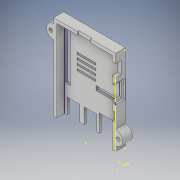
# Autodesk Inventor part: Oberteil_fertig2
Saved by Autodesk Inventor 2017 (Build 210142000, 142)
## iProperties
Part Number: Oberteil_fertig2
Material: Generisch
Document SubType Name: Modeling
Designer: Fynn
Density: 1 g/cm^3
Appearance: Vorgabe
Author: Fynn
Autodesk Inventor part; units mm, degrees
ref_plane "YZ Plane" through (0, 0, 0) normal (1, 0, 0) x (0, 1, 0)
ref_plane "XZ Plane" through (0, 0, 0) normal (0, 1, 0) x (-1, 0, 0)
ref_plane "XY Plane" through (0, 0, 0) normal (0, 0, 1) x (1, 0, 0)
sketch "Skizze1" plane through (0, 0, 0) normal (0, 1, 0) x (-1, 0, 0)
  line L0 (64.3291, 15.6705) -> (64.3291, 102.6705)
  line L1 (64.3291, 102.6705) -> (5.4791, 102.6705)
  line L2 (61.5291, 32.1705) -> (48.0291, 32.1705)
  line L3 (48.0291, 32.1705) -> (48.0291, 15.6705)
  line L4 (61.5291, 15.6705) -> (61.5291, 32.1705)
  line L5 (43.5291, 32.1705) -> (30.0291, 32.1705)
  line L6 (30.0291, 32.1705) -> (30.0291, 15.6705)
  line L7 (30.0291, 15.6705) -> (30.7791, 15.6705)
  line L8 (43.5291, 15.6705) -> (43.5291, 32.1705)
  line L9 (27.5291, 34.6705) -> (9.9291, 34.6705)
  line L10 (9.9291, 34.6705) -> (9.9291, 15.6705)
  line L11 (27.5291, 15.6705) -> (27.5291, 34.6705)
  line L12 (30.7791, 58.1705) -> (5.4791, 58.1705)
  line L13 (5.4791, 53.6705) -> (30.7791, 53.6705)
  line L14 (30.7791, 53.6705) -> (30.7791, 58.1705)
  line L15 (5.4791, 102.6705) -> (5.4791, 58.1705)
  line L16 (5.4791, 53.6705) -> (5.4791, 15.6705)
  line L17 (43.5291, 15.6705) -> (48.0291, 15.6705)
  line L18 (61.5291, 15.6705) -> (64.3291, 15.6705)
  line L19 (50.9791, 78.7705) -> (30.9791, 78.7705)
  line L20 (30.9791, 78.7705) -> (30.9791, 76.7705)
  line L21 (30.9791, 76.7705) -> (50.9791, 76.7705)
  line L22 (50.9791, 76.7705) -> (50.9791, 78.7705)
  line L23 (50.9791, 73.7705) -> (30.9791, 73.7705)
  line L24 (30.9791, 73.7705) -> (30.9791, 71.7705)
  line L25 (30.9791, 71.7705) -> (50.9791, 71.7705)
  line L26 (50.9791, 71.7705) -> (50.9791, 73.7705)
  line L27 (50.9791, 68.7705) -> (30.9791, 68.7705)
  line L28 (30.9791, 68.7705) -> (30.9791, 66.7705)
  line L29 (30.9791, 66.7705) -> (50.9791, 66.7705)
  line L30 (50.9791, 66.7705) -> (50.9791, 68.7705)
  line L31 (50.9791, 63.7705) -> (30.9791, 63.7705)
  line L32 (30.9791, 63.7705) -> (30.9791, 61.7705)
  line L33 (30.9791, 61.7705) -> (50.9791, 61.7705)
  line L34 (50.9791, 61.7705) -> (50.9791, 63.7705)
  line L35 (5.4791, 15.6705) -> (9.9291, 15.6705)
  line L36 (27.5291, 15.6705) -> (30.0291, 15.6705)
  line L37 (5.4791, 58.1705) -> (5.4791, 63.7705)
  line L38 (62.9791, 94.6705) -> (57.4791, 94.6705)
  line L39 (57.4791, 94.6705) -> (57.4791, 41.6705)
  line L40 (57.4791, 41.6705) -> (62.9791, 41.6705)
  line L41 (62.9791, 41.6705) -> (62.9791, 94.6705)
  dimension "d2" = 13.5
  dimension "d3" = 13.5
  dimension "d45" = 2.8
  dimension "d46" = 4.5
  dimension "d47" = 2.5
  dimension "d49" = 42.5
  dimension "d51" = 49
  dimension "d60" = 53
  dimension "d61" = 8
  dimension "d62" = 5.5
  dimension "d63" = 1.35
  dimension "d70" = 87
  dimension "d71" = 87
  dimension "d107" = 4.45
  dimension "d108" = 38
  dimension "d110" = 17.6
  dimension "d141" = 25.3
  dimension "d142" = 19
  constraints: 84 end point, 22 parallel, 13 horizontal, 13 perpendicular, 4 point on line
  measures "d2" distance of L2.start L2.end
  measures "d3" distance of L5.start L5.end
  measures "d45" distance of L4.start L0.start
  measures "d46" distance of L8.start L3.end
  measures "d47" distance of L11.start L6.end
  measures "d49" distance between parallel lines of L35 L12
  measures "d51" distance between parallel lines of L1 L13
  measures "d60" distance of L40.end L38.start
  measures "d61" distance between parallel lines of L1 L38
  measures "d62" distance of L38.start L38.end
  measures "d63" distance between parallel lines of L0 L41
  measures "d70" distance of L0.start L0.end
  measures "d71" distance of L16.end L1.end
  measures "d107" distance of L16.end L10.end
  measures "d108" distance of L13.start L16.end
  measures "d110" distance of L9.start L9.end
  measures "d141" distance between parallel lines of L14 L15
  measures "d142" distance between parallel lines of L13 L9
sketch "Skizze2" plane through (0, 0, 0) normal (0, 1, 0) x (-1, 0, 0)
  point P0 (0, 0)
extrude "Extrusion1" add sketch "Skizze1" along normal blind 3.5 contours L18 L4 L2 L3 L17 L8 L5 L6 L36 L11 L9 L10 L35 L16 L13 L14 L12 L15 L1 L0 | L41 L40 L39 L38
sketch "Skizze3" plane through (0, 0, 0) normal (0, -1, 0) x (1, 0, 0)
  line L0 (-9.9291, 15.6705) -> (-5.4791, 15.6705) projected
  line L1 (-64.3291, 102.6705) -> (-5.4791, 102.6705) projected
  line L2 (-5.4791, 15.6705) -> (-5.4791, 102.6705)
  line L3 (-5.4791, 102.6705) -> (-64.3291, 102.6705)
  line L4 (-64.3291, 102.6705) -> (-64.3291, 15.6705)
  point P0 (0, 0)
  constraints: 6 end point, 1 collinear, 1 perpendicular
sketch "Skizze4" plane through (0, 0, 0) normal (0, -1, 0) x (1, 0, 0)
  line L0 (-30.7791, 53.6705) -> (-5.4791, 53.6705) projected
  line L1 (-5.4791, 53.6705) -> (-5.4791, 15.6705) projected
  line L2 (-5.4791, 15.6705) -> (-5.4791, 102.6705)
  line L3 (-64.3291, 102.6705) -> (-5.4791, 102.6705) projected
  line L4 (-5.4791, 102.6705) -> (-64.3291, 102.6705)
  line L5 (-61.5291, 15.6705) -> (-64.3291, 15.6705) projected
  line L6 (-64.3291, 102.6705) -> (-64.3291, 15.6705)
  point P0 (0, 0)
  point P1 (-5.4791, 68.3705)
  point P2 (-5.4791, 63.3705)
  constraints: 6 end point, 2 perpendicular, 1 vertical, 1 other
sketch "Skizze5" plane through (0, 3.5, 0) normal (0, 1, 0) x (1, 0, 0)
  point P0 (0, 0)
sketch "Skizze6" plane through (0, 3.5, 0) normal (0, 1, 0) x (1, 0, 0)
  point P0 (0, 0)
sketch "Skizze7" plane through (0, 3.5, 0) normal (0, 1, 0) x (1, 0, 0)
  point P0 (0, 0)
sketch "Skizze8" plane through (0, 3.5, 0) normal (0, 1, 0) x (1, 0, 0)
  point P0 (0, 0)
sketch "Skizze9" plane through (0, 3.5, 0) normal (0, 1, 0) x (1, 0, 0)
  point P0 (0, 0)
sketch "Skizze10" plane through (0, 3.5, 0) normal (0, 1, 0) x (1, 0, 0)
  line L0 (-57.8291, -44.6705) -> (-63.3291, -44.6705)
  line L1 (-63.3291, -44.6705) -> (-63.3291, -95.6705)
  line L2 (-63.3291, -95.6705) -> (-57.8291, -95.6705)
  line L3 (-57.8291, -95.6705) -> (-57.8291, -44.6705)
  line L4 (-64.3291, -102.6705) -> (-5.4791, -102.6705) projected
  line L5 (-64.3291, -15.6705) -> (-64.3291, -102.6705) projected
  point P0 (0, 0)
  dimension "d64" = 51
  dimension "d65" = 5.5
  dimension "d66" = 7
  dimension "d67" = 1
  constraints: 8 end point, 2 parallel, 1 horizontal, 1 perpendicular
  measures "d64" distance of L2.end L0.start
  measures "d65" distance of L0.start L0.end
  measures "d66" distance between parallel lines of L4 L2
  measures "d67" distance between parallel lines of L5 L1
extrude "Extrusion2" cut sketch "Skizze10" against normal through all
sketch "Skizze11" plane through (0, 3.5, 0) normal (0, 1, 0) x (1, 0, 0)
  line L0 (-64.3291, -102.6705) -> (-64.3291, -15.6705) projected
  line L1 (-64.3291, -15.6705) -> (-64.3291, -102.6705) projected
  line L2 (-64.3291, -15.6705) -> (-67.8291, -15.6705)
  line L3 (-67.8291, -15.6705) -> (-67.8291, -106.1705)
  line L4 (-67.8291, -106.1705) -> (-1.9791, -106.1705)
  line L5 (-1.9791, -106.1705) -> (-1.9791, -15.6705)
  line L6 (-1.9791, -15.6705) -> (-5.4791, -15.6705)
  line L7 (-64.3291, -102.6705) -> (-5.4791, -102.6705) projected
  line L8 (-5.4791, -102.6705) -> (-64.3291, -102.6705)
  line L9 (-64.3291, -102.6705) -> (-64.3291, -15.6705)
  line L10 (-64.3291, -15.6705) -> (-64.3291, -102.6705)
  line L11 (-5.4791, -53.6705) -> (-5.4791, -15.6705) projected
  line L12 (-5.4791, -102.6705) -> (-5.4791, -15.6705)
  line L13 (-5.4791, -15.6705) -> (-1.9791, -15.6705)
  point P0 (0, 0)
  dimension "d77" = 3.5
  dimension "d78" = 3.5
  dimension "d79" = 3.5
  constraints: 20 end point, 6 perpendicular, 2 horizontal, 1 point on line, 1 vertical
  measures "d77" distance of L0.end L2.end
  measures "d78" distance of L5.end L6.end
  measures "d79" distance between parallel lines of L7 L4
sketch "Skizze12" plane through (0, 0, 0) normal (0, -1, 0) x (1, 0, 0)
  line L0 (-5.4791, 15.6705) -> (-9.9291, 15.6705) projected
  line L1 (-5.4791, 102.6705) -> (-5.4791, 58.1705) projected
  line L2 (-5.4791, 15.6705) -> (-5.4791, 102.6705)
  line L3 (-5.4791, 102.6705) -> (-64.3291, 102.6705)
  line L4 (-64.3291, 102.6705) -> (-64.3291, 15.6705)
  point P0 (0, 0)
  constraints: 6 end point, 2 perpendicular, 1 vertical
extrude "Extrusion3" add sketch "Skizze11" against normal blind 11.6
sketch "Skizze13" plane through (0, 3.5, 0) normal (0, 1, 0) x (1, 0, 0)
  line L0 (-67.8291, -15.6705) -> (-67.8291, -106.1705) projected
  arc A0 (-67.8291, -85.6705) -> (-67.8291, -100.6705) centre (-67.8291, -93.1705) ccw
  arc A1 (-67.8291, -21.1705) -> (-67.8291, -36.1705) centre (-67.8291, -28.6705) ccw
  arc A2 (-1.9791, -36.1705) -> (-1.9791, -21.1705) centre (-1.9791, -28.6705) ccw
  arc A3 (-1.9791, -100.6705) -> (-1.9791, -85.6705) centre (-1.9791, -93.1705) ccw
  line L1 (-67.8291, -106.1705) -> (-1.9791, -106.1705) projected
  line L2 (-1.9791, -15.6705) -> (-9.9291, -15.6705) projected
  line L3 (-1.9791, -106.1705) -> (-1.9791, -15.6705) projected
  point P0 (0, 0)
  dimension "d82" = 15
  dimension "d83" = 15
  dimension "d84" = 15
  dimension "d85" = 15
  dimension "d86" = 13
  dimension "d87" = 13
  dimension "d88" = 13
  dimension "d89" = 13
  constraints: 10 point on line, 8 point on circle, 4 centre point
  measures "d82" diameter of A0
  measures "d83" diameter of A1
  measures "d84" diameter of A2
  measures "d85" diameter of A3
  measures "d86" distance from line of A3.centre L1
  measures "d87" distance from line of L2 A2.centre
  measures "d88" distance from line of L1 A0.centre
  measures "d89" distance of A1.centre L0.start
extrude "Extrusion4" add sketch "Skizze13" against normal blind 11.6
sketch "Skizze14" plane through (0, 3.5, 0) normal (0, 1, 0) x (1, 0, 0)
  arc A0 (-1.9791, -36.1705) -> (-1.9791, -21.1705) centre (-1.9791, -28.6705) ccw projected
  arc A1 (-1.9791, -100.6705) -> (-1.9791, -85.6705) centre (-1.9791, -93.1705) ccw projected
  arc A2 (-67.8291, -85.6705) -> (-67.8291, -100.6705) centre (-67.8291, -93.1705) ccw projected
  arc A3 (-67.8291, -21.1705) -> (-67.8291, -36.1705) centre (-67.8291, -28.6705) ccw projected
  point P0 (0, 0)
  point P1 (-70.8291, -93.1705)
  point P2 (-70.8291, -28.6705)
  point P3 (1.0209, -93.1705)
  point P4 (1.0209, -28.6705)
  dimension "d92" = 0
  dimension "d93" = 3
  dimension "d94" = 0
  dimension "d95" = 3
  dimension "d96" = 0
  dimension "d97" = 3
  dimension "d98" = 0
  dimension "d99" = 3
  measures "d92" vertical distance of point (1.021, -28.671) A0.centre
  measures "d93" distance of A0.centre point (1.021, -28.671)
  measures "d94" vertical distance of A1.centre point (1.021, -93.171)
  measures "d95" distance of A1.centre point (1.021, -93.171)
  measures "d96" vertical distance of A2.centre point (-70.829, -93.171)
  measures "d97" distance of A2.centre point (-70.829, -93.171)
  measures "d98" vertical distance of A3.centre point (-70.829, -28.671)
  measures "d99" distance of point (-70.829, -28.671) A3.centre
hole "Bohrung1" at (-70.8291, 3.5, 28.6705) at (1.0209, 3.5, 28.6705) at (1.0209, 3.5, 93.1705) at (-70.8291, 3.5, 93.1705) direction (0, -1, 0) diameter 4 end through all
sketch "Skizze15" plane through (0, 3.5, 0) normal (0, 1, 0) x (1, 0, 0)
  point P0 (0, 0)
sketch "Skizze16" plane through (0, 3.5, 0) normal (0, 1, 0) x (1, 0, 0)
  point P0 (0, 0)
sketch "Skizze17" plane through (-9.9291, 0, 15.6705) normal (0, 0, -1) x (-1, 0, 0)
  point P0 (-9.9291, 0)
sketch "Skizze18" plane through (0, 3.5, 0) normal (0, 1, 0) x (1, 0, 0)
  line L0 (-1.9791, -106.1705) -> (-1.9791, -100.6705) projected
  line L1 (-1.9791, -103.4205) -> (11.4811, -103.4205)
  line L2 (11.4811, -103.4205) -> (11.4811, -74.2753)
  line L3 (11.4811, -74.2753) -> (-1.9791, -74.2753)
  line L4 (-1.9791, -74.2753) -> (-1.9791, -103.4205)
  line L5 (-67.8291, -36.1705) -> (-67.8291, -85.6705) projected
  line L6 (-67.8291, -38.1575) -> (-77.5027, -38.1575)
  line L7 (-77.5027, -38.1575) -> (-77.5027, -17.1859)
  line L8 (-77.5027, -17.1859) -> (-67.8291, -17.1859)
  line L9 (-67.8291, -17.1859) -> (-67.8291, -38.1575)
  point P0 (0, 0)
  constraints: 16 end point, 4 parallel, 2 horizontal, 2 perpendicular, 1 midpoint, 1 point on line
extrude "Extrusion5" cut sketch "Skizze18" against normal blind 20
sketch "Skizze19" plane through (0, 3.5, 0) normal (0, 1, 0) x (1, 0, 0)
  point P0 (0, 0)
sketch "Skizze20" plane through (-67.8291, 3.5, 106.1705) normal (0, 0, 1) x (1, 0, 0)
  point P0 (67.8291, -3.5)
sketch "Skizze21" plane through (-67.8291, 3.5, 106.1705) normal (0, 0, 1) x (1, 0, 0)
  line L0 (65.85, -11.6) -> (0, -11.6) projected
  line L1 (26.425, -11.6) -> (39.425, -11.6)
  line L2 (39.425, -11.6) -> (39.425, -10.1)
  line L3 (39.425, -10.1) -> (26.425, -10.1)
  line L4 (26.425, -10.1) -> (26.425, -11.6)
  line L5 (65.85, 0) -> (65.85, -11.6) projected
  point P0 (67.8291, -3.5)
  dimension "d113" = 13
  dimension "d114" = 1.5
  dimension "d115" = 26.425
  constraints: 8 end point, 2 parallel, 1 horizontal, 1 perpendicular, 1 point on line
  measures "d113" distance of L2.end L3.end
  measures "d114" distance of L1.end L2.end
  measures "d115" distance from line of L5 L1.end
extrude "Extrusion6" cut sketch "Skizze21" along normal mid plane 20
sketch "Skizze22" plane through (0, 3.5, 0) normal (0, 1, 0) x (1, 0, 0)
  point P0 (0, 0)
sketch "Skizze23" plane through (0, 3.5, 0) normal (0, 1, 0) x (1, 0, 0)
  point P0 (0, 0)
sketch "Skizze24" plane through (-1.9791, -8.1, 106.1705) normal (1, 0, 0) x (0, 0, -1)
  line L0 (5.5, 0) -> (20.5, 0) projected
  line L1 (7.3789, 0) -> (15, 0)
  line L2 (90.5, 0) -> (3.5, 0) projected
  line L3 (30, 0) -> (45, 0)
  line L4 (45, 0) -> (45, 7.8)
  line L5 (45, 7.8) -> (30, 7.8)
  line L6 (30, 7.8) -> (30, 0)
  line L7 (9.4, 0) -> (22.4, 0)
  line L8 (22.4, 0) -> (22.4, 6)
  line L9 (22.4, 6) -> (9.4, 6)
  line L10 (9.4, 6) -> (9.4, 0)
  line L11 (0, 11.6) -> (0, 0) projected
  point P0 (106.1705, 8.1)
  point P1 (15.9, 6)
  dimension "d118" = 15
  dimension "d119" = 13
  dimension "d120" = 6
  dimension "d121" = 15.9
  dimension "d122" = 7.8
  dimension "d123" = 45
  constraints: 18 end point, 4 parallel, 3 horizontal, 3 point on line, 2 perpendicular, 1 midpoint
  measures "d118" distance of L4.end L5.end
  measures "d119" distance of L8.end L9.end
  measures "d120" distance of L9.end L7.start
  measures "d121" distance from line of L11 point (15.9, 6)
  measures "d122" distance of L3.end L4.end
  measures "d123" distance between parallel lines of L11 L4
sketch "Skizze25" plane through (0, -8.1, 0) normal (0, -1, 0) x (1, 0, 0)
  point P0 (0, 0)
extrude "Extrusion7" cut sketch "Skizze24" against normal blind 20
sketch "Skizze26" plane through (-1.9791, -8.1, 106.1705) normal (1, 0, 0) x (0, 0, -1)
  line L0 (20.5, 0) -> (90.5, 0) projected
  line L1 (44.8289, 0) -> (47.7248, 0)
  point P0 (106.1705, 8.1)
  constraints: 2 end point, 2 point on line
sketch "Skizze27" plane through (-1.9791, -8.1, 106.1705) normal (1, 0, 0) x (0, 0, -1)
  line L0 (20.5, 0) -> (90.5, 0) projected
  line L1 (45.0921, 0) -> (47.3, 0)
  line L2 (47.3, 0) -> (47.3, 10.1)
  line L3 (10.5, 8.1) -> (61.5, 8.1) projected
  line L4 (47.3, 10.1) -> (27.7, 10.1)
  line L5 (27.7, 10.1) -> (27.7, 0)
  line L6 (27.7, 0) -> (30, 0)
  line L7 (30, 0) -> (30, 7.8) projected
  line L8 (30, 0) -> (30, 7.8)
  line L9 (45, 7.8) -> (45, 0) projected
  line L10 (30, 7.8) -> (45, 7.8)
  line L11 (45, 7.8) -> (45, 0)
  line L12 (45, 0) -> (47.3, 0)
  line L13 (70, 0) -> (70, 11.6) projected
  point P0 (106.1705, 8.1)
  dimension "d126" = 2.3
  dimension "d127" = 2.3
  dimension "d128" = 2.3
  constraints: 18 end point, 5 perpendicular, 3 point on line, 2 collinear, 1 horizontal
  measures "d126" distance between parallel lines of L2 L9
  measures "d127" distance between parallel lines of L4 L10
  measures "d128" distance between parallel lines of L5 L7
extrude "Extrusion8" cut sketch "Skizze27" against normal blind 1.8 contours L5 L3 L2 L0 L9 L10 L7 | L5 L4 L2 L3
sketch "Skizze28" plane through (-1.9791, -8.1, 106.1705) normal (1, 0, 0) x (0, 0, -1)
  point P0 (106.1705, 8.1)
sketch "Skizze29" plane through (0, -8.1, 0) normal (0, -1, 0) x (1, 0, 0)
  point P0 (0, 0)
sketch "Skizze30" plane through (0, 3.5, 0) normal (0, 1, 0) x (1, 0, 0)
  point P0 (0, 0)
sketch "Skizze31" plane through (0, -8.1, 0) normal (0, -1, 0) x (1, 0, 0)
  line L0 (-5.4791, 15.6705) -> (-5.4791, 53.6705) projected
  line L1 (-5.4791, 51.6705) -> (-2.9791, 51.6705)
  line L2 (-2.9791, 51.6705) -> (-2.9791, 42.6705)
  line L3 (-2.9791, 42.6705) -> (-5.4791, 42.6705)
  line L4 (-5.4791, 15.6705) -> (-1.9791, 15.6705) projected
  point P0 (0, 0)
  dimension "d131" = 36
  dimension "d132" = 27
  dimension "d133" = 2.5
  constraints: 6 end point, 3 perpendicular, 2 point on line
  measures "d131" distance between parallel lines of L4 L1
  measures "d132" distance between parallel lines of L4 L3
  measures "d133" distance of L2.end L3.end
sketch "Skizze32" plane through (-5.4791, 3.5, 53.6705) normal (-1, 0, 0) x (0, 0, 1)
  point P0 (-53.6705, -3.5)
extrude "Extrusion9" cut sketch "Skizze31" against normal blind 8.1
sketch "Skizze33" plane through (0, -8.1, 0) normal (0, -1, 0) x (1, 0, 0)
  line L0 (-67.8291, 106.1705) -> (-1.9791, 106.1705) projected
  line L1 (-41.3093, 106.1705) -> (-45.3093, 106.1705)
  line L2 (-45.3093, 106.1705) -> (-45.3093, 102.6705)
  line L3 (-5.4791, 102.6705) -> (-64.3291, 102.6705) projected
  line L4 (-41.3093, 102.6705) -> (-41.3093, 106.1705)
  point P0 (0, 0)
  constraints: 6 end point, 4 point on line, 2 perpendicular
sketch "Skizze34" plane through (-41.4041, -8.1, 106.1705) normal (1, 0, 0) x (0, 0, -1)
  point P0 (106.1705, 8.1)
extrude "Extrusion10" cut sketch "Skizze33" against normal blind 1.5
sketch "Skizze35" plane through (0, 3.5, 0) normal (0, 1, 0) x (1, 0, 0)
  point P0 (0, 0)
sketch "Skizze36" plane through (0, 3.5, 0) normal (0, 1, 0) x (1, 0, 0)
  point P0 (0, 0)
sketch "Skizze37" plane through (-9.9291, 0, 34.6705) normal (0, 0, -1) x (-1, 0, 0)
  point P0 (-9.9291, 0)
sketch "Skizze38" plane through (0, 3.5, 0) normal (0, 1, 0) x (1, 0, 0)
  line L0 (-78.4732, -10.8186) -> (12.9519, -10.8186)
  line L1 (12.9519, -10.8186) -> (12.9519, -110.1672)
  line L2 (12.9519, -110.1672) -> (-78.4732, -110.1672)
  line L3 (-78.4732, -110.1672) -> (-78.4732, -10.8186)
  point P0 (0, 0)
  constraints: 8 end point, 2 parallel, 1 horizontal, 1 perpendicular
extrude "Extrusion11" cut sketch "Skizze38" against normal blind 1
sketch "Skizze39" plane through (0, -8.1, 0) normal (0, -1, 0) x (1, 0, 0)
  point P0 (0, 0)
sketch "Skizze40" plane through (-28.4041, -8.1, 106.1705) normal (0, 0, 1) x (1, 0, 0)
  point P0 (28.4041, 8.1)
sketch "Skizze41" plane through (0, 2.5, 0) normal (0, 1, 0) x (1, 0, 0)
  point P0 (0, 0)
sketch "Skizze42" plane through (0, 2.5, 0) normal (0, 1, 0) x (1, 0, 0)
  point P0 (0, 0)
sketch "Skizze43" plane through (-30.0291, 0, 32.1705) normal (0, 0, -1) x (-1, 0, 0)
  point P0 (-30.0291, 0)
sketch "Skizze44" plane through (-9.9291, 0, 34.6705) normal (0, 0, -1) x (-1, 0, 0)
  point P0 (-9.9291, 0)
sketch "Skizze45" plane through (0, 2.5, 0) normal (0, 1, 0) x (1, 0, 0)
  point P0 (0, 0)
sketch "Skizze46" plane through (-28.4041, -6.6, 102.6705) normal (0, -1, 0) x (1, 0, 0)
  line L0 (0, 0) -> (-16.9052, 0) projected
  line L1 (-16.9052, 0) -> (-16.9052, 3.5) projected
  line L2 (-16.9052, 3.5) -> (0, 3.5) projected
  line L3 (-16.9052, 3.5) -> (-13.9052, 3.5)
  line L4 (-13.9052, 3.5) -> (-13.9052, 0)
  line L5 (-13.9052, 0) -> (-16.9052, 0)
  line L6 (-16.9052, 0) -> (-16.9052, 3.5)
  point P0 (28.4041, -102.6705)
  dimension "d143" = 3
  dimension "d144" = 3.5
  constraints: 8 end point, 2 parallel, 1 horizontal, 1 perpendicular
  measures "d143" distance of L4.end L5.end
  measures "d144" distance of L3.end L4.end
extrude "Extrusion12" add sketch "Skizze46" along normal blind 1.5
